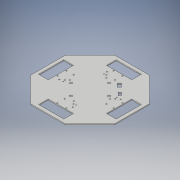
# Autodesk Inventor part: Base
Saved by Autodesk Inventor 2019 (Build 230136000, 136)
## iProperties
Created: 2019-03-08
Part Number: Base
Material: Generic
Document SubType Name: Modeling
Designer: jonas
Density: 1 g/cm^3
Appearance: Default
Author: jonas
Autodesk Inventor part; units mm, degrees
ref_plane "YZ Plane" through (0, 0, 0) normal (1, 0, 0) x (0, 1, 0)
ref_plane "XZ Plane" through (0, 0, 0) normal (0, 1, 0) x (-1, 0, 0)
ref_plane "XY Plane" through (0, 0, 0) normal (0, 0, 1) x (1, 0, 0)
sketch "Sketch2" plane through (0, 0, 0) normal (0, 1, 0) x (-1, 0, 0)
  line L0 (-54, -130.3675) -> (-130.3675, -54)
  line L1 (-130.3675, -54) -> (-130.3675, 54)
  line L2 (-130.3675, 54) -> (-54, 130.3675)
  line L3 (-54, 130.3675) -> (54, 130.3675)
  line L4 (54, 130.3675) -> (130.3675, 54)
  line L5 (130.3675, 54) -> (130.3675, -54)
  line L6 (130.3675, -54) -> (54, -130.3675)
  line L7 (54, -130.3675) -> (-54, -130.3675)
  line L8 (41175.9013, 0) -> (-41175.9013, 0) projected
  line L9 (-39, -120.3675) -> (39, -120.3675)
  line L10 (39, -120.3675) -> (39, -90.3675)
  line L11 (39, -90.3675) -> (-39, -90.3675)
  line L12 (-39, -90.3675) -> (-39, -120.3675)
  line L13 (90.3675, -39) -> (120.3675, -39)
  line L14 (90.3675, 39) -> (90.3675, -39)
  line L15 (120.3675, -39) -> (120.3675, 39)
  line L16 (120.3675, 39) -> (90.3675, 39)
  line L17 (39, 90.3675) -> (39, 120.3675)
  line L18 (-39, 90.3675) -> (39, 90.3675)
  line L19 (39, 120.3675) -> (-39, 120.3675)
  line L20 (-39, 120.3675) -> (-39, 90.3675)
  line L21 (-90.3675, 39) -> (-120.3675, 39)
  line L22 (-90.3675, -39) -> (-90.3675, 39)
  line L23 (-120.3675, 39) -> (-120.3675, -39)
  line L24 (-120.3675, -39) -> (-90.3675, -39)
  circle A0 centre (-13.775, -86.8675) radius 1.6
  line L25 (0, -2693.5297) -> (0, 2693.5297) projected
  circle A1 centre (-13.775, -64.5175) radius 1.6
  circle A2 centre (13.775, -86.8675) radius 1.6
  circle A3 centre (13.775, -64.5175) radius 1.6
  circle A4 centre (86.8675, -13.775) radius 1.6
  circle A5 centre (86.8675, 13.775) radius 1.6
  circle A6 centre (64.5175, -13.775) radius 1.6
  circle A7 centre (64.5175, 13.775) radius 1.6
  circle A8 centre (13.775, 86.8675) radius 1.6
  circle A9 centre (-13.775, 86.8675) radius 1.6
  circle A10 centre (13.775, 64.5175) radius 1.6
  circle A11 centre (-13.775, 64.5175) radius 1.6
  circle A12 centre (-86.8675, 13.775) radius 1.6
  circle A13 centre (-86.8675, -13.775) radius 1.6
  circle A14 centre (-64.5175, 13.775) radius 1.6
  circle A15 centre (-64.5175, -13.775) radius 1.6
  line L26 (-14.2258, -50.4297) -> (-15.64, -49.0154)
  line L27 (-15.64, -49.0154) -> (-9.9831, -43.3586)
  line L28 (-9.9831, -43.3586) -> (-8.5689, -44.7728)
  line L29 (-8.5689, -44.7728) -> (-14.2258, -50.4297)
  line L30 (-41175.9013, 0) -> (41175.9013, 0)
  circle A16 centre (20.9157, -74.2574) radius 1.6
  line L31 (0, 2693.5297) -> (0, -2693.5297)
  line L32 (-48.6843, -48.6843) -> (48.6843, 48.6843)
  line L33 (-48.6843, -48.6843) -> (89.0157, -48.6843) construction
  line L34 (16.6877, -16.6877) -> (-16.6877, 16.6877)
  line L35 (-50.4297, -14.2258) -> (-49.0154, -15.64)
  line L36 (-49.0154, -15.64) -> (-43.3586, -9.9831)
  line L37 (-43.3586, -9.9831) -> (-44.7728, -8.5689)
  line L38 (-44.7728, -8.5689) -> (-50.4297, -14.2258)
  line L39 (50.4297, 14.2258) -> (49.0154, 15.64)
  line L40 (49.0154, 15.64) -> (43.3586, 9.9831)
  line L41 (43.3586, 9.9831) -> (44.7728, 8.5689)
  line L42 (44.7728, 8.5689) -> (50.4297, 14.2258)
  line L43 (9.9831, 43.3586) -> (8.5689, 44.7728)
  line L44 (14.2258, 50.4297) -> (15.64, 49.0154)
  line L45 (15.64, 49.0154) -> (9.9831, 43.3586)
  line L46 (8.5689, 44.7728) -> (14.2258, 50.4297)
  line L47 (-32.0673, -65.4427) -> (-42.6739, -54.8361)
  line L48 (-42.6739, -54.8361) -> (-36.3099, -48.4722)
  line L49 (-36.3099, -48.4722) -> (-25.7033, -59.0788)
  line L50 (-25.7033, -59.0788) -> (-32.0673, -65.4427)
  line L51 (-56.9575, -40.5526) -> (-65.4427, -32.0673)
  line L52 (-65.4427, -32.0673) -> (-60.1394, -26.764)
  line L53 (-60.1394, -26.764) -> (-51.6542, -35.2493)
  line L54 (-51.6542, -35.2493) -> (-56.9575, -40.5526)
  line L55 (20.1657, -61.8405) -> (20.1657, -64.5905) construction
  line L56 (19.4157, -62.5905) -> (19.4157, -63.8405)
  line L57 (20.9157, -63.8405) -> (20.9157, -62.5905)
  arc A17 (20.9157, -62.5905) -> (19.4157, -62.5905) centre (20.1657, -62.5905) ccw
  arc A18 (19.4157, -63.8405) -> (20.9157, -63.8405) centre (20.1657, -63.8405) ccw
  arc A19 (62.5905, 20.9157) -> (62.5905, 19.4157) centre (62.5905, 20.1657) ccw
  line L58 (63.8405, 20.9157) -> (62.5905, 20.9157)
  line L59 (62.5905, 19.4157) -> (63.8405, 19.4157)
  arc A20 (63.8405, 19.4157) -> (63.8405, 20.9157) centre (63.8405, 20.1657) ccw
  line L60 (61.8405, 20.1657) -> (64.5905, 20.1657) construction
  arc A21 (-20.9157, 62.5905) -> (-19.4157, 62.5905) centre (-20.1657, 62.5905) ccw
  line L61 (-20.9157, 63.8405) -> (-20.9157, 62.5905)
  line L62 (-19.4157, 62.5905) -> (-19.4157, 63.8405)
  arc A22 (-19.4157, 63.8405) -> (-20.9157, 63.8405) centre (-20.1657, 63.8405) ccw
  line L63 (-20.1657, 61.8405) -> (-20.1657, 64.5905) construction
  arc A23 (-62.5905, -20.9157) -> (-62.5905, -19.4157) centre (-62.5905, -20.1657) ccw
  line L64 (-63.8405, -20.9157) -> (-62.5905, -20.9157)
  line L65 (-62.5905, -19.4157) -> (-63.8405, -19.4157)
  arc A24 (-63.8405, -19.4157) -> (-63.8405, -20.9157) centre (-63.8405, -20.1657) ccw
  line L66 (-61.8405, -20.1657) -> (-64.5905, -20.1657) construction
  circle A25 centre (0, -949.3978) radius 1.6
  circle A26 centre (949.3978, 0) radius 1.6
  circle A27 centre (0, 949.3978) radius 1.6
  circle A28 centre (-949.3978, 0) radius 1.6
  circle A29 centre (5.8021, -56.3462) radius 1.6
  circle A30 centre (74.2574, 20.9157) radius 1.6
  circle A31 centre (56.3462, 5.8021) radius 1.6
  circle A32 centre (-20.9157, 74.2574) radius 1.6
  circle A33 centre (-5.8021, 56.3462) radius 1.6
  circle A34 centre (-74.2574, -20.9157) radius 1.6
  circle A35 centre (-56.3462, -5.8021) radius 1.6
  point P0 (0, 0)
  point P1 (0, 0)
  point P2 (0, 0)
  point P3 (0, 0)
  point P4 (0, 0)
  point P5 (0, 0)
  point P6 (0, 0)
  point P7 (0, 0)
  point P8 (20.1657, -63.2155)
  point P9 (63.2155, 20.1657)
  point P10 (-20.1657, 63.2155)
  point P11 (-63.2155, -20.1657)
  dimension "d5" = 10
  dimension "d6" = 30
  dimension "d7" = 15
  dimension "d8" = 15
  dimension "d11" = 360
  dimension "d13" = 78
  dimension "d14" = 13.775
  dimension "d16" = 3.5
  dimension "d18" = 22.35
  dimension "d21" = 360
  dimension "d24" = 2
  dimension "d25" = 8
  dimension "d29" = 3.2
  dimension "d41" = 3.2
  dimension "d48" = 137.7
  dimension "d49" = 45
  dimension "d50" = 47.2
  dimension "d51" = 23.6
  dimension "d52" = 9
  dimension "d53" = 15
  dimension "d56" = 68.95
  dimension "d57" = 23.6
  dimension "d58" = 68.95
  dimension "d59" = 23.6
  dimension "d60" = 7.5
  dimension "d61" = 12
  dimension "d62" = 2.75
  dimension "d63" = 1.5
  dimension "d66" = 360
  dimension "d70" = 3.2
  dimension "d73" = 360
  dimension "d83" = 3.2
  dimension "d86" = 360
  constraints: 138 end point, 36 centre point, 24 point on circle, 18 symmetric about line, 13 parallel, 9 point on line, 6 midpoint, 6 perpendicular, 4 coincident, 4 tangent, 2 horizontal, 1 equal length, 1 equal radius, 170 other
  measures "d5" distance between parallel lines of L9 L7
  measures "d6" distance between parallel lines of L11 L9
  measures "d7" distance from line of L0.start L12
  measures "d8" distance from line of L6.end L10
  measures "d13" distance between parallel lines of L12 L10
  measures "d14" distance from line of L25 A0.centre
  measures "d16" distance from line of A0.centre L11
  measures "d18" distance of A1.centre A0.centre
  measures "d24" distance between parallel lines of L27 L29
  measures "d25" distance between parallel lines of L28 L26
  measures "d29" diameter of A3
  measures "d41" diameter of A16
  measures "d48" distance of L32.start L32.end
  measures "d49" angle of L33 L32
  measures "d50" distance of L34.start L34.end
  measures "d51" distance between parallel lines of L32 L27
  measures "d52" distance between parallel lines of L49 L47
  measures "d53" distance between parallel lines of L48 L50
  measures "d56" distance between parallel lines of L34 L47
  measures "d57" distance between parallel lines of L32 L50
  measures "d58" distance between parallel lines of L51 L34
  measures "d59" distance between parallel lines of L52 L32
  measures "d60" distance between parallel lines of L51 L53
  measures "d61" distance between parallel lines of L52 L54
  measures "d62" distance of L55.start L55.end
  measures "d63" diameter of A18
  measures "d70" diameter of A25
  measures "d83" diameter of A29
extrude "Extrusion5" add sketch "Sketch2" along normal blind 3 contours L0 L1 L8 L23 L24 L22 L25 L11 L12 L9 L7 | L25 L9 L10 L11 L8 L14 L13 L15 L5 L6 L7 | L1 L2 L3 L25 L19 L20 L18 L8 L22 L21 L23 | L8 L15 L16 L14 L25 L18 L17 L19 L3 L4 L5
equation "\"d8\" = d7"
body "Solid5"
